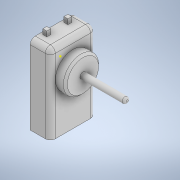
# Autodesk Inventor part: dc
Saved by Autodesk Inventor 2022 (Build 260153070, 153G)
## iProperties
Created: 2021-07-26
Part Number: dc
Material: Generic
Document SubType Name: Modeling
Designer: AKASH ARYAN
Density: 1 g/cm^3
Appearance: Default
Author: AKASH ARYAN
Autodesk Inventor part; units mm, degrees
ref_plane "YZ Plane" through (0, 0, 0) normal (1, 0, 0) x (0, 1, 0)
ref_plane "XZ Plane" through (0, 0, 0) normal (0, 1, 0) x (-1, 0, 0)
ref_plane "XY Plane" through (0, 0, 0) normal (0, 0, 1) x (1, 0, 0)
sketch "Sketch1" plane through (0, 0, 0) normal (1, 0, 0) x (0, 1, 0)
  line L0 (0, 0) -> (-78.6, 0)
  line L1 (-78.6, 0) -> (-78.6, -45)
  line L2 (-78.6, -45) -> (0, -45)
  line L3 (0, -45) -> (0, 0)
  dimension "d0" = 78.6
  dimension "d1" = 45
  constraints: 8 end point, 2 parallel, 1 horizontal, 1 perpendicular
  measures "d0" distance of L2.end L1.end
  measures "d1" distance of L1.end L0.end
extrude "Extrusion1" add sketch "Sketch1" along normal blind 20
sketch "Sketch2" plane through (20, 0, 0) normal (1, 0, 0) x (0, 0, -1)
  circle A0 centre (22.5, -27.8) radius 17.5
  line L0 (45, -78.6) -> (45, 0) projected
  line L1 (0, -78.6) -> (45, -78.6) projected
  point P0 (0, 0)
  dimension "d4" = 35
  dimension "d5" = 22.5
  dimension "d6" = 50.8
  constraints: 1 centre point
  measures "d4" diameter of A0
  measures "d5" distance from line of L0 A0.centre
  measures "d6" distance from line of L1 A0.centre
extrude "Extrusion2" add sketch "Sketch2" along normal blind 10
sketch "Sketch3" plane through (30, -27.8, -22.5) normal (1, 0, 0) x (0, 0, -1)
  circle A0 centre (0, 0) radius 3
  point P0 (-22.5, 27.8)
  dimension "d9" = 6
  constraints: 1 centre point
  measures "d9" diameter of A0
extrude "Extrusion3" add sketch "Sketch3" along normal blind 44
fillet "Fillet1" radius 5 2 edges at (10, 0, 0) (10, 0, -45)
sketch "Sketch4" plane through (0, 0, -5) normal (0, 1, 0) x (1, 0, 0)
  line L0 (6.488, 30) -> (2.488, 30)
  line L1 (2.488, 30) -> (2.488, 26)
  line L2 (2.488, 26) -> (6.488, 26)
  line L3 (6.488, 26) -> (6.488, 30)
  line L4 (6.488, 9) -> (2.488, 9)
  line L5 (2.488, 9) -> (2.488, 5)
  line L6 (2.488, 5) -> (6.488, 5)
  line L7 (6.488, 5) -> (6.488, 9)
  line L8 (0, 35) -> (20, 35) projected
  line L9 (20, 0) -> (0, 0) projected
  point P0 (0, -5)
  dimension "d13" = 4
  dimension "d14" = 4
  dimension "d15" = 4
  dimension "d16" = 4
  dimension "d17" = 5
  dimension "d18" = 9
  constraints: 16 end point, 4 parallel, 2 horizontal, 2 perpendicular
  measures "d13" distance of L2.end L1.end
  measures "d14" distance of L1.end L0.end
  measures "d15" distance of L6.end L5.end
  measures "d16" distance of L5.end L4.end
  measures "d17" distance from line of L8 L0.end
  measures "d18" distance between parallel lines of L9 L4
extrude "Extrusion4" add sketch "Sketch4" along normal blind 5
chamfer "Chamfer1" distance 2 angle 45 1 edges at (30, -27.8, -5)
fillet "Fillet2" radius 5 5 edges at (20, -1.4645, -1.4645) (20, -41.8, 0) (20, -1.4645, -43.5355) (20, -41.8, -45) (20, 0, -22.5)
fillet "Fillet3" radius 2 1 edges at (74, -27.8, -19.5)
sketch "Sketch5" plane through (30, -27.8, -22.5) normal (1, 0, 0) x (0, 0, -1)
  point P0 (-22.5, 27.8)
body "Solid1"
